Autodesk Fusion 360 part; units mm, degrees
(part 3 of 7)
  spline S687 degree 3 poles (51.2491, 62.2155) (51.339, 62.0596) (51.4081, 61.8927) (51.4547, 61.7189) knots 0 0 0 0 1 1 1 1
  spline S688 degree 3 poles (83.1324, 72.6381) (82.8108, 72.6437) (82.5167, 72.8204) (82.3608, 73.1016) knots 0 0 0 0 1 1 1 1
  spline S689 degree 3 poles (42.3721, 73.5812) (42.197, 73.8508) (42.1791, 74.1934) (42.3251, 74.4798) knots 0 0 0 0 1 1 1 1
  spline S690 degree 3 poles (108.782, 65.514) (108.9517, 65.7864) (108.9635, 66.1286) (108.813, 66.4121) knots 0 0 0 0 1 1 1 1
  spline S691 degree 3 poles (111.5839, 53.8372) (111.8201, 53.6007) (112.1405, 53.4678) (112.4748, 53.4677) knots 0 0 0 0 1 1 1 1
  spline S692 degree 3 poles (111.5839, 55.619) (111.3476, 55.3827) (111.2149, 55.0622) (111.2149, 54.7281) knots 0 0 0 0 1 1 1 1
  line L235 (43.0795, 74.9702) -> (44.388, 75.0385)
  spline S693 degree 3 poles (51.525, 61.1856) (51.525, 61.0055) (51.5014, 60.8262) (51.4547, 60.6523) knots 0 0 0 0 1 1 1 1
  line L236 (44.4665, 75.039) -> (44.4665, 75.039)
  spline S694 degree 3 poles (113.4943, 55.4686) (113.4167, 55.5755) (113.3227, 55.6695) (113.2158, 55.7471) knots 0 0 0 0 1 1 1 1
  spline S695 degree 3 poles (49.998, 63.1751) (50.172, 63.1286) (50.3391, 63.0594) (50.4951, 62.9694) knots 0 0 0 0 1 1 1 1
  spline S696 degree 3 poles (51.4547, 60.6523) (51.4081, 60.4785) (51.339, 60.3115) (51.2491, 60.1557) knots 0 0 0 0 1 1 1 1
  spline S697 degree 3 poles (51.4547, 61.7189) (51.5014, 61.5449) (51.525, 61.3656) (51.525, 61.1856) knots 0 0 0 0 1 1 1 1
  spline S698 degree 3 poles (113.6731, 55.1172) (113.6323, 55.243) (113.572, 55.3616) (113.4943, 55.4686) knots 0 0 0 0 1 1 1 1
  line L237 (112.4748, 55.9879) -> (112.4748, 55.9879)
  spline S699 degree 3 poles (45.237, 73.7316) (45.0911, 73.4449) (44.8032, 73.258) (44.482, 73.2412) knots 0 0 0 0 1 1 1 1
  line L238 (43.0826, 79.1343) -> (43.0826, 79.1343)
  spline S700 degree 3 poles (70.73, 75.2436) (71.0515, 75.2435) (71.3486, 75.072) (71.5093, 74.7935) knots 0 0 0 0 1 1 1 1
  spline S701 degree 3 poles (82.3769, 74.0013) (82.5425, 74.2768) (82.8425, 74.4431) (83.1639, 74.4375) knots 0 0 0 0 1 1 1 1
  line L239 (69.42, 75.2436) -> (69.42, 75.2436)
  spline S702 degree 3 poles (43.1741, 73.1724) (42.8529, 73.1556) (42.5472, 73.3114) (42.3721, 73.5812) knots 0 0 0 0 1 1 1 1
  line L240 (108.0518, 66.8896) -> (106.7428, 66.9356)
  spline S703 degree 3 poles (68.6407, 73.8938) (68.4801, 74.1722) (68.4801, 74.5151) (68.6407, 74.7935) knots 0 0 0 0 1 1 1 1
  spline S704 degree 3 poles (42.3251, 74.4798) (42.4709, 74.7663) (42.7585, 74.9533) (43.0795, 74.9702) knots 0 0 0 0 1 1 1 1
  spline S705 degree 3 poles (113.0685, 70.4573) (113.4027, 70.4575) (113.7232, 70.5904) (113.9594, 70.8268) knots 0 0 0 0 1 1 1 1
  spline S706 degree 3 poles (114.3284, 71.7177) (114.3283, 71.8499) (114.3073, 71.9812) (114.2664, 72.1069) knots 0 0 0 0 1 1 1 1
  spline S707 degree 3 poles (125.4285, 67.8353) (125.1002, 68.1635) (124.9158, 68.6087) (124.9159, 69.0729) knots 0 0 0 0 1 1 1 1
  spline S708 degree 3 poles (108.6016, 70.1256) (108.7576, 70.2155) (108.9011, 70.3255) (109.0285, 70.4527) knots 0 0 0 0 1 1 1 1
  line L241 (114.2307, 72.1771) -> (112.0303, 72.2541)
  spline S709 degree 3 poles (108.105, 69.9199) (108.2788, 69.9665) (108.4458, 70.0356) (108.6016, 70.1256) knots 0 0 0 0 1 1 1 1
  spline S710 degree 3 poles (109.5612, 71.3761) (109.6079, 71.5501) (109.6315, 71.7294) (109.6315, 71.9095) knots 0 0 0 0 1 1 1 1
  spline S711 degree 3 poles (109.6315, 71.9095) (109.6278, 72.0545) (109.6087, 72.1988) (109.5747, 72.3399) knots 0 0 0 0 1 1 1 1
  spline S712 degree 3 poles (112.1771, 70.8268) (112.4134, 70.5903) (112.7341, 70.4573) (113.0685, 70.4573) knots 0 0 0 0 1 1 1 1
  line L242 (109.0982, 72.3565) -> (109.1287, 73.2355)
  spline S713 degree 3 poles (102.0749, 73.3616) (101.7407, 73.3616) (101.4203, 73.2288) (101.184, 72.9926) knots 0 0 0 0 1 1 1 1
  spline S714 degree 3 poles (109.0383, 54.9198) (109.0383, 55.0999) (109.0146, 55.2792) (108.968, 55.4531) knots 0 0 0 0 1 1 1 1
  spline S715 degree 3 poles (103.3347, 72.1017) (103.3348, 72.2338) (103.314, 72.3651) (103.2733, 72.4908) knots 0 0 0 0 1 1 1 1
  line L243 (102.0749, 73.3616) -> (102.0749, 73.3616)
  spline S716 degree 3 poles (103.0944, 72.8422) (103.0166, 72.9491) (102.9225, 73.0431) (102.8154, 73.1207) knots 0 0 0 0 1 1 1 1
  spline S717 degree 3 poles (88.1264, 72.2505) (87.8053, 72.2553) (87.506, 72.0887) (87.3409, 71.8133) knots 0 0 0 0 1 1 1 1
  spline S718 degree 3 poles (108.968, 55.4531) (108.9214, 55.6269) (108.8523, 55.7939) (108.7623, 55.9497) knots 0 0 0 0 1 1 1 1
  spline S719 degree 3 poles (101.4816, 56.3719) (101.1475, 56.3719) (100.827, 56.2392) (100.5907, 56.0029) knots 0 0 0 0 1 1 1 1
  line L244 (106.9784, 56.9801) -> (106.9784, 56.9801)
  spline S720 degree 3 poles (126.6656, 67.3227) (126.2016, 67.3227) (125.7566, 67.5071) (125.4285, 67.8353) knots 0 0 0 0 1 1 1 1
  spline S721 degree 3 poles (124.9159, 69.0729) (124.9159, 69.537) (125.1003, 69.982) (125.4285, 70.3101) knots 0 0 0 0 1 1 1 1
  spline S722 degree 3 poles (101.184, 71.2103) (101.4203, 70.974) (101.7407, 70.8413) (102.0749, 70.8413) knots 0 0 0 0 1 1 1 1
  spline S723 degree 3 poles (102.4645, 73.2995) (102.3387, 73.3405) (102.2072, 73.3615) (102.0749, 73.3616) knots 0 0 0 0 1 1 1 1
  spline S724 degree 3 poles (127.9033, 67.8353) (127.575, 67.507) (127.1298, 67.3226) (126.6656, 67.3227) knots 0 0 0 0 1 1 1 1
  spline S725 degree 3 poles (100.815, 72.1017) (100.8149, 71.7674) (100.9476, 71.4467) (101.184, 71.2103) knots 0 0 0 0 1 1 1 1
  line L245 (88.0949, 70.4511) -> (89.4048, 70.4279)
  spline S726 degree 3 poles (107.5717, 73.9693) (107.0253, 73.9694) (106.5013, 73.7525) (106.1149, 73.3662) knots 0 0 0 0 1 1 1 1
  spline S727 degree 3 poles (102.9658, 71.2103) (103.2022, 71.4467) (103.3349, 71.7674) (103.3347, 72.1017) knots 0 0 0 0 1 1 1 1
  spline S728 degree 3 poles (106.1149, 73.3662) (105.7287, 72.9798) (105.5118, 72.4558) (105.5119, 71.9095) knots 0 0 0 0 1 1 1 1
  spline S729 degree 3 poles (87.3409, 71.8133) (87.176, 71.5381) (87.1701, 71.1959) (87.3254, 70.9152) knots 0 0 0 0 1 1 1 1
  spline S730 degree 3 poles (102.8154, 73.1207) (102.7085, 73.1984) (102.5901, 73.2587) (102.4645, 73.2995) knots 0 0 0 0 1 1 1 1
  spline S731 degree 3 poles (87.3254, 70.9152) (87.4808, 70.6344) (87.774, 70.4576) (88.0949, 70.4511) knots 0 0 0 0 1 1 1 1
  spline S732 degree 3 poles (108.968, 54.3865) (109.0146, 54.5604) (109.0383, 54.7397) (109.0383, 54.9198) knots 0 0 0 0 1 1 1 1
  line L246 (126.6656, 70.8227) -> (126.6656, 70.8227)
  spline S733 degree 3 poles (114.2664, 72.1069) (114.2552, 72.1306) (114.2433, 72.1541) (114.2307, 72.1771) knots 0 0 0 0 1 1 1 1
  spline S734 degree 3 poles (102.0749, 70.8413) (102.409, 70.8413) (102.7295, 70.974) (102.9658, 71.2103) knots 0 0 0 0 1 1 1 1
  spline S735 degree 3 poles (109.3556, 70.8795) (109.4455, 71.0354) (109.5147, 71.2023) (109.5612, 71.3761) knots 0 0 0 0 1 1 1 1
  line L247 (89.4359, 72.2278) -> (88.1264, 72.2505)
  spline S736 degree 3 poles (90.2058, 71.7637) (90.0503, 72.0447) (89.7569, 72.2215) (89.4359, 72.2278) knots 0 0 0 0 1 1 1 1
  spline S737 degree 3 poles (89.4048, 70.4279) (89.7257, 70.4232) (90.0248, 70.5898) (90.1898, 70.8651) knots 0 0 0 0 1 1 1 1
  spline S738 degree 3 poles (108.105, 73.8995) (107.931, 73.946) (107.7517, 73.9694) (107.5717, 73.9693) knots 0 0 0 0 1 1 1 1
  spline S739 degree 3 poles (101.184, 72.9926) (100.9477, 72.7563) (100.815, 72.4358) (100.815, 72.1017) knots 0 0 0 0 1 1 1 1
  spline S740 degree 3 poles (113.9594, 70.8268) (114.1957, 71.0631) (114.3284, 71.3836) (114.3284, 71.7177) knots 0 0 0 0 1 1 1 1
  line L248 (109.5747, 72.3399) -> (109.0982, 72.3565)
  spline S741 degree 3 poles (103.2733, 72.4908) (103.2325, 72.6166) (103.1721, 72.7352) (103.0944, 72.8422) knots 0 0 0 0 1 1 1 1
  spline S742 degree 3 poles (108.0084, 56.7037) (107.8525, 56.7938) (107.6856, 56.8631) (107.5118, 56.9099) knots 0 0 0 0 1 1 1 1
  spline S743 degree 3 poles (128.4159, 69.0729) (128.4159, 68.6087) (128.2315, 68.1635) (127.9033, 67.8353) knots 0 0 0 0 1 1 1 1
  spline S744 degree 3 poles (125.4285, 70.3101) (125.7566, 70.6382) (126.2016, 70.8226) (126.6656, 70.8227) knots 0 0 0 0 1 1 1 1
  spline S745 degree 3 poles (90.1898, 70.8651) (90.3551, 71.1403) (90.3612, 71.4828) (90.2058, 71.7637) knots 0 0 0 0 1 1 1 1
  spline S746 degree 3 poles (101.0258, 68.7856) (100.8557, 68.5131) (100.8437, 68.1707) (100.9943, 67.887) knots 0 0 0 0 1 1 1 1
  spline S747 degree 3 poles (101.8191, 69.2088) (101.4981, 69.2194) (101.1958, 69.0581) (101.0258, 68.7856) knots 0 0 0 0 1 1 1 1
  spline S748 degree 3 poles (108.4352, 56.3766) (108.3078, 56.5038) (108.1643, 56.6137) (108.0084, 56.7037) knots 0 0 0 0 1 1 1 1
  spline S749 degree 3 poles (109.0285, 70.4527) (109.1557, 70.5801) (109.2656, 70.7236) (109.3556, 70.8795) knots 0 0 0 0 1 1 1 1
  spline S750 degree 3 poles (100.9943, 67.887) (101.145, 67.6035) (101.4352, 67.4218) (101.756, 67.41) knots 0 0 0 0 1 1 1 1
  spline S751 degree 3 poles (109.0285, 73.3662) (108.9011, 73.4934) (108.7576, 73.6034) (108.6016, 73.6933) knots 0 0 0 0 1 1 1 1
  spline S752 degree 3 poles (106.1149, 70.4527) (106.5013, 70.0664) (107.0253, 69.8495) (107.5717, 69.8496) knots 0 0 0 0 1 1 1 1
  spline S753 degree 3 poles (107.5118, 56.9099) (107.3378, 56.9565) (107.1585, 56.9801) (106.9784, 56.9801) knots 0 0 0 0 1 1 1 1
  spline S754 degree 3 poles (111.8081, 71.7177) (111.8081, 71.3836) (111.9408, 71.0631) (112.1771, 70.8268) knots 0 0 0 0 1 1 1 1
  spline S755 degree 3 poles (108.7623, 55.9497) (108.6724, 56.1057) (108.5624, 56.2492) (108.4352, 56.3766) knots 0 0 0 0 1 1 1 1
  spline S756 degree 3 poles (108.6016, 73.6933) (108.4458, 73.7835) (108.2788, 73.8528) (108.105, 73.8995) knots 0 0 0 0 1 1 1 1
  spline S757 degree 3 poles (112.0303, 72.2541) (111.9155, 72.0951) (111.8394, 71.9114) (111.8081, 71.7177) knots 0 0 0 0 1 1 1 1
  spline S758 degree 3 poles (105.5119, 71.9095) (105.5118, 71.3631) (105.7287, 70.8391) (106.1149, 70.4527) knots 0 0 0 0 1 1 1 1
  spline S759 degree 3 poles (109.1287, 73.2355) (109.097, 73.2804) (109.0636, 73.324) (109.0285, 73.3662) knots 0 0 0 0 1 1 1 1
  spline S760 degree 3 poles (107.5717, 69.8496) (107.7518, 69.8496) (107.9311, 69.8733) (108.105, 69.9199) knots 0 0 0 0 1 1 1 1
  spline S761 degree 3 poles (99.6285, 38.1224) (99.6285, 38.4565) (99.7612, 38.777) (99.9975, 39.0133) knots 0 0 0 0 1 1 1 1
  spline S762 degree 3 poles (52.0955, 38.372) (52.1288, 38.5277) (52.1203, 38.6894) (52.0707, 38.8407) knots 0 0 0 0 1 1 1 1
  spline S763 degree 3 poles (105.918, 65.6137) (106.0687, 65.3303) (106.359, 65.1485) (106.6798, 65.1367) knots 0 0 0 0 1 1 1 1
  spline S764 degree 3 poles (34.5209, 42.8735) (34.5311, 42.7409) (34.5942, 42.618) (34.6961, 42.5324) knots 0 0 0 0 1 1 1 1
  line L249 (39.5454, 42.8115) -> (39.6456, 41.6658)
  line L250 (13.8684, 45.3834) -> (13.8684, 45.3834)
  spline S765 degree 3 poles (101.7793, 37.2315) (101.5431, 36.995) (101.2226, 36.8621) (100.8884, 36.862) knots 0 0 0 0 1 1 1 1
  spline S766 degree 3 poles (9.1416, 27.9669) (9.2946, 27.9668) (9.447, 27.9467) (9.5948, 27.907) knots 0 0 0 0 1 1 1 1
  spline S767 degree 3 poles (10.6572, 27.092) (10.7336, 26.9596) (10.7924, 26.8176) (10.8319, 26.6698) knots 0 0 0 0 1 1 1 1
  line L251 (51.2702, 39.25) -> (49.9623, 39.1812)
  spline S768 degree 3 poles (10.017, 27.7323) (10.1493, 27.6559) (10.2711, 27.5624) (10.3792, 27.4543) knots 0 0 0 0 1 1 1 1
  spline S769 degree 3 poles (10.8319, 26.6698) (10.8716, 26.5221) (10.8918, 26.3697) (10.8918, 26.2166) knots 0 0 0 0 1 1 1 1
  spline S770 degree 3 poles (99.9975, 39.0133) (100.2338, 39.2495) (100.5542, 39.3823) (100.8884, 39.3822) knots 0 0 0 0 1 1 1 1
  spline S771 degree 3 poles (49.2094, 38.6908) (49.1958, 38.5844) (49.2014, 38.4764) (49.2259, 38.372) knots 0 0 0 0 1 1 1 1
  spline S772 degree 3 poles (9.1416, 24.4669) (8.6775, 24.467) (8.2325, 24.6514) (7.9044, 24.9795) knots 0 0 0 0 1 1 1 1
  spline S773 degree 3 poles (7.9044, 24.9795) (7.5763, 25.3076) (7.3919, 25.7526) (7.3918, 26.2166) knots 0 0 0 0 1 1 1 1
  spline S774 degree 3 poles (7.3918, 26.2166) (7.3918, 26.6809) (7.5762, 27.1261) (7.9044, 27.4543) knots 0 0 0 0 1 1 1 1
  spline S775 degree 3 poles (29.0101, 30.3962) (28.8745, 30.1052) (28.5941, 29.9085) (28.2742, 29.88) knots 0 0 0 0 1 1 1 1
  line L252 (33.892, 44.3246) -> (34.4335, 43.8698)
  spline S776 degree 3 poles (100.8884, 39.3822) (101.0207, 39.3823) (101.1522, 39.3616) (101.278, 39.3208) knots 0 0 0 0 1 1 1 1
  line L253 (34.4335, 43.8698) -> (34.5209, 42.8735)
  spline S777 degree 3 poles (49.2259, 38.372) (49.2014, 38.4764) (49.1958, 38.5844) (49.2094, 38.6908) knots 0 0 0 0 1 1 1 1
  spline S778 degree 3 poles (103.0655, 67.364) (103.3863, 67.3536) (103.6884, 67.5149) (103.8582, 67.7872) knots 0 0 0 0 1 1 1 1
  spline S779 degree 3 poles (34.6961, 42.5324) (34.798, 42.447) (34.9301, 42.4062) (35.0624, 42.4193) knots 0 0 0 0 1 1 1 1
  spline S780 degree 3 poles (51.2702, 39.25) (51.591, 39.2661) (51.896, 39.1101) (52.0707, 38.8407) knots 0 0 0 0 1 1 1 1
  spline S781 degree 3 poles (49.2094, 38.6908) (49.355, 38.9768) (49.6418, 39.1637) (49.9623, 39.1812) knots 0 0 0 0 1 1 1 1
  spline S782 degree 3 poles (10.8918, 26.2166) (10.8917, 25.7526) (10.7073, 25.3076) (10.3792, 24.9795) knots 0 0 0 0 1 1 1 1
  spline S783 degree 3 poles (102.1483, 38.1224) (102.1483, 37.7882) (102.0155, 37.4678) (101.7793, 37.2315) knots 0 0 0 0 1 1 1 1
  spline S784 degree 3 poles (10.3792, 24.9795) (10.051, 24.6512) (9.6058, 24.4668) (9.1416, 24.4669) knots 0 0 0 0 1 1 1 1
  spline S785 degree 3 poles (101.6289, 39.1414) (101.736, 39.0638) (101.8301, 38.9698) (101.908, 38.8629) knots 0 0 0 0 1 1 1 1
  line L254 (42.2108, 41.8901) -> (42.5183, 38.372)
  spline S786 degree 3 poles (101.278, 39.3208) (101.4037, 39.2798) (101.5221, 39.2192) (101.6289, 39.1414) knots 0 0 0 0 1 1 1 1
  spline S787 degree 3 poles (7.9044, 27.4543) (8.2325, 27.7824) (8.6775, 27.9668) (9.1416, 27.9669) knots 0 0 0 0 1 1 1 1
  line L255 (28.2742, 29.88) -> (26.9694, 29.7658)
  line L256 (49.2259, 38.372) -> (52.0955, 38.372)
  spline S788 degree 3 poles (52.0707, 38.8407) (51.896, 39.1101) (51.591, 39.2661) (51.2702, 39.25) knots 0 0 0 0 1 1 1 1
  spline S789 degree 3 poles (28.1962, 31.6763) (28.4894, 31.6758) (28.764, 31.5325) (28.9321, 31.2923) knots 0 0 0 0 1 1 1 1
  spline S790 degree 3 poles (99.9975, 37.2315) (99.7612, 37.4678) (99.6285, 37.7882) (99.6285, 38.1224) knots 0 0 0 0 1 1 1 1
  spline S791 degree 3 poles (28.9321, 31.2923) (29.1162, 31.029) (29.1459, 30.6874) (29.0101, 30.3962) knots 0 0 0 0 1 1 1 1
  spline S792 degree 3 poles (26.1545, 30.1461) (25.9702, 30.4094) (25.9403, 30.7509) (26.0759, 31.0422) knots 0 0 0 0 1 1 1 1
  spline S793 degree 3 poles (28.1177, 31.6732) (28.1438, 31.6753) (28.17, 31.6764) (28.1962, 31.6763) knots 0 0 0 0 1 1 1 1
  spline S794 degree 3 poles (106.7428, 66.9356) (106.4218, 66.9462) (106.1195, 66.7849) (105.9496, 66.5124) knots 0 0 0 0 1 1 1 1
  line L257 (103.128, 69.1628) -> (101.8191, 69.2088)
  spline S795 degree 3 poles (14.7614, 44.1065) (14.897, 44.3978) (14.8671, 44.7393) (14.6828, 45.0026) knots 0 0 0 0 1 1 1 1
  spline S796 degree 3 poles (14.6828, 45.0026) (14.4987, 45.2657) (14.1884, 45.4109) (13.8684, 45.3834) knots 0 0 0 0 1 1 1 1
  spline S797 degree 3 poles (26.9694, 29.7658) (26.6493, 29.738) (26.3388, 29.883) (26.1545, 30.1461) knots 0 0 0 0 1 1 1 1
  line L258 (35.0624, 42.4193) -> (39.5454, 42.8115)
  line L259 (100.8884, 39.3822) -> (100.8884, 39.3822)
  line L260 (106.6798, 65.1367) -> (107.9887, 65.0907)
  spline S798 degree 3 poles (10.3792, 27.4543) (10.4873, 27.3462) (10.5808, 27.2244) (10.6572, 27.092) knots 0 0 0 0 1 1 1 1
  line L261 (9.1416, 27.9669) -> (9.1416, 27.9669)
  spline S799 degree 3 poles (105.9496, 66.5124) (105.7795, 66.2399) (105.7674, 65.8974) (105.918, 65.6137) knots 0 0 0 0 1 1 1 1
  spline S800 degree 3 poles (9.5948, 27.907) (9.7425, 27.8675) (9.8845, 27.8087) (10.017, 27.7323) knots 0 0 0 0 1 1 1 1
  spline S801 degree 3 poles (103.8898, 68.6854) (103.7392, 68.969) (103.4489, 69.151) (103.128, 69.1628) knots 0 0 0 0 1 1 1 1
  line L262 (5.5077, 35.7706) -> (5.5077, 35.7706)
  spline S802 degree 3 poles (101.908, 38.8629) (101.9856, 38.7559) (102.046, 38.6373) (102.0868, 38.5115) knots 0 0 0 0 1 1 1 1
  spline S803 degree 3 poles (103.8582, 67.7872) (104.0282, 68.0596) (104.0402, 68.4018) (103.8898, 68.6854) knots 0 0 0 0 1 1 1 1
  line L263 (101.756, 67.41) -> (103.0655, 67.364)
  spline S804 degree 3 poles (49.9623, 39.1812) (49.6418, 39.1637) (49.355, 38.9768) (49.2094, 38.6908) knots 0 0 0 0 1 1 1 1
  line L264 (39.6456, 41.6658) -> (42.2108, 41.8901)
  line L265 (49.9623, 39.1812) -> (51.2702, 39.25)
  spline S805 degree 3 poles (100.8884, 36.862) (100.5542, 36.8621) (100.2337, 36.995) (99.9975, 37.2315) knots 0 0 0 0 1 1 1 1
  line L266 (42.5183, 38.372) -> (49.2259, 38.372)
  spline S806 degree 3 poles (102.0868, 38.5115) (102.1275, 38.3858) (102.1483, 38.2545) (102.1483, 38.1224) knots 0 0 0 0 1 1 1 1
  spline S807 degree 3 poles (26.7141, 33.2012) (26.38, 33.2012) (26.0595, 33.3339) (25.8232, 33.5702) knots 0 0 0 0 1 1 1 1
  line L267 (106.8022, 31.1114) -> (105.4933, 31.1574)
  spline S808 degree 3 poles (25.8232, 35.352) (26.0594, 35.5884) (26.3799, 35.7214) (26.7141, 35.7215) knots 0 0 0 0 1 1 1 1
  spline S809 degree 3 poles (7.0233, 34.8957) (7.0998, 34.7632) (7.1585, 34.6213) (7.198, 34.4735) knots 0 0 0 0 1 1 1 1
  spline S810 degree 3 poles (7.198, 34.4735) (7.2377, 34.3259) (7.2578, 34.1737) (7.258, 34.0208) knots 0 0 0 0 1 1 1 1
  spline S811 degree 3 poles (6.7453, 32.7832) (6.417, 32.4551) (5.9718, 32.2709) (5.5077, 32.2711) knots 0 0 0 0 1 1 1 1
  spline S812 degree 3 poles (100.5695, 33.4307) (100.2487, 33.4424) (99.9585, 33.6242) (99.8078, 33.9076) knots 0 0 0 0 1 1 1 1
  line L268 (100.6321, 35.2295) -> (100.6321, 35.2295)
  spline S813 degree 3 poles (3.7579, 34.0208) (3.7579, 34.485) (3.9423, 34.9302) (4.2705, 35.2585) knots 0 0 0 0 1 1 1 1
  spline S814 degree 3 poles (98.6616, 20.925) (98.8355, 20.8784) (99.0024, 20.8093) (99.1583, 20.7193) knots 0 0 0 0 1 1 1 1
  spline S815 degree 3 poles (68.7818, 18.5267) (68.7818, 18.9909) (68.9662, 19.4361) (69.2945, 19.7643) knots 0 0 0 0 1 1 1 1
  spline S816 degree 3 poles (99.1583, 20.7193) (99.3142, 20.6294) (99.4577, 20.5194) (99.5851, 20.3922) knots 0 0 0 0 1 1 1 1
  spline S817 degree 3 poles (102.6717, 33.8079) (102.5018, 33.5354) (102.1995, 33.3741) (101.8785, 33.3847) knots 0 0 0 0 1 1 1 1
  line L269 (26.8123, 31.559) -> (28.1177, 31.6732)
  spline S818 degree 3 poles (26.7141, 35.7215) (26.8465, 35.7214) (26.9779, 35.7005) (27.1038, 35.6595) knots 0 0 0 0 1 1 1 1
  line L270 (26.7141, 35.7215) -> (26.7141, 35.7215)
  spline S819 degree 3 poles (25.4543, 34.4611) (25.4542, 34.7952) (25.587, 35.1157) (25.8232, 35.352) knots 0 0 0 0 1 1 1 1
  line L271 (105.5558, 32.9563) -> (106.8653, 32.9103)
  spline S820 degree 3 poles (104.7626, 32.5331) (104.9325, 32.8056) (105.2348, 32.9668) (105.5558, 32.9563) knots 0 0 0 0 1 1 1 1
  spline S821 degree 3 poles (7.258, 34.0208) (7.258, 33.5566) (7.0736, 33.1114) (6.7453, 32.7832) knots 0 0 0 0 1 1 1 1
  spline S822 degree 3 poles (99.8394, 34.8063) (100.0092, 35.0786) (100.3113, 35.2399) (100.6321, 35.2295) knots 0 0 0 0 1 1 1 1
  spline S823 degree 3 poles (5.5077, 32.2711) (5.0437, 32.271) (4.5987, 32.4552) (4.2705, 32.7832) knots 0 0 0 0 1 1 1 1
  spline S824 degree 3 poles (27.1038, 35.6595) (27.2294, 35.6186) (27.3478, 35.5583) (27.4546, 35.4807) knots 0 0 0 0 1 1 1 1
  spline S825 degree 3 poles (27.974, 34.4611) (27.974, 34.329) (27.9533, 34.1977) (27.9125, 34.072) knots 0 0 0 0 1 1 1 1
  spline S826 degree 3 poles (5.9609, 35.7112) (6.1085, 35.6716) (6.2502, 35.6129) (6.3826, 35.5365) knots 0 0 0 0 1 1 1 1
  spline S827 degree 3 poles (4.2705, 32.7832) (3.9423, 33.1114) (3.7579, 33.5566) (3.7579, 34.0208) knots 0 0 0 0 1 1 1 1
  spline S828 degree 3 poles (102.7033, 34.706) (102.8537, 34.4225) (102.8417, 34.0802) (102.6717, 33.8079) knots 0 0 0 0 1 1 1 1
  line L272 (105.5558, 32.9563) -> (105.5558, 32.9563)
  spline S829 degree 3 poles (69.2945, 19.7643) (69.6226, 20.0925) (70.0676, 20.2769) (70.5316, 20.277) knots 0 0 0 0 1 1 1 1
  spline S830 degree 3 poles (25.8232, 33.5702) (25.587, 33.8065) (25.4542, 34.127) (25.4543, 34.4611) knots 0 0 0 0 1 1 1 1
  spline S831 degree 3 poles (27.4546, 35.4807) (27.5617, 35.4029) (27.6559, 35.3087) (27.7337, 35.2016) knots 0 0 0 0 1 1 1 1
  spline S832 degree 3 poles (101.9416, 35.1835) (102.2625, 35.1717) (102.5527, 34.9897) (102.7033, 34.706) knots 0 0 0 0 1 1 1 1
  spline S833 degree 3 poles (5.5077, 35.7706) (5.6607, 35.7707) (5.8131, 35.7507) (5.9609, 35.7112) knots 0 0 0 0 1 1 1 1
  spline S834 degree 3 poles (4.2705, 35.2585) (4.5987, 35.5864) (5.0437, 35.7706) (5.5077, 35.7706) knots 0 0 0 0 1 1 1 1
  line L273 (70.5316, 20.277) -> (70.5316, 20.277)
  spline S835 degree 3 poles (27.7337, 35.2016) (27.8113, 35.0948) (27.8717, 34.9764) (27.9125, 34.8507) knots 0 0 0 0 1 1 1 1
  spline S836 degree 3 poles (27.7337, 33.7206) (27.6559, 33.6137) (27.5617, 33.5197) (27.4546, 33.442) knots 0 0 0 0 1 1 1 1
  spline S837 degree 3 poles (107.6285, 32.4333) (107.7793, 32.1495) (107.7673, 31.8067) (107.597, 31.5342) knots 0 0 0 0 1 1 1 1
  spline S838 degree 3 poles (99.5851, 20.3922) (99.7123, 20.2648) (99.8223, 20.1213) (99.9122, 19.9654) knots 0 0 0 0 1 1 1 1
  spline S839 degree 3 poles (100.1184, 19.4687) (100.1649, 19.2948) (100.1883, 19.1155) (100.1882, 18.9354) knots 0 0 0 0 1 1 1 1
  spline S840 degree 3 poles (100.1184, 18.4021) (100.0717, 18.2283) (100.0023, 18.0613) (99.9122, 17.9055) knots 0 0 0 0 1 1 1 1
  spline S841 degree 3 poles (98.1283, 20.9953) (98.3084, 20.9952) (98.4877, 20.9716) (98.6616, 20.925) knots 0 0 0 0 1 1 1 1
  spline S842 degree 3 poles (99.9122, 17.9055) (99.8223, 17.7496) (99.7123, 17.6061) (99.5851, 17.4787) knots 0 0 0 0 1 1 1 1
  spline S843 degree 3 poles (99.5851, 17.4787) (99.4577, 17.3515) (99.3142, 17.2415) (99.1583, 17.1516) knots 0 0 0 0 1 1 1 1
  spline S844 degree 3 poles (26.0759, 31.0422) (26.2115, 31.3336) (26.4922, 31.5305) (26.8123, 31.559) knots 0 0 0 0 1 1 1 1
  spline S845 degree 3 poles (98.6616, 16.9454) (98.4877, 16.8987) (98.3084, 16.8751) (98.1283, 16.8751) knots 0 0 0 0 1 1 1 1
  spline S846 degree 3 poles (99.1583, 17.1516) (99.0024, 17.0614) (98.8355, 16.9921) (98.6616, 16.9454) knots 0 0 0 0 1 1 1 1
  line L274 (100.6321, 35.2295) -> (101.9416, 35.1835)
  spline S847 degree 3 poles (27.4546, 33.442) (27.3478, 33.3642) (27.2294, 33.3037) (27.1038, 33.2627) knots 0 0 0 0 1 1 1 1
  spline S848 degree 3 poles (99.9122, 19.9654) (100.0023, 19.8095) (100.0717, 19.6426) (100.1184, 19.4687) knots 0 0 0 0 1 1 1 1
  spline S849 degree 3 poles (100.1882, 18.9354) (100.1883, 18.7554) (100.1649, 18.5761) (100.1184, 18.4021) knots 0 0 0 0 1 1 1 1
  spline S850 degree 3 poles (27.9125, 34.072) (27.8717, 33.9462) (27.8114, 33.8276) (27.7337, 33.7206) knots 0 0 0 0 1 1 1 1
  spline S851 degree 3 poles (99.8078, 33.9076) (99.6572, 34.1914) (99.6692, 34.5338) (99.8394, 34.8063) knots 0 0 0 0 1 1 1 1
  spline S852 degree 3 poles (27.9125, 34.8507) (27.9533, 34.7249) (27.9741, 34.5934) (27.974, 34.4611) knots 0 0 0 0 1 1 1 1
  spline S853 degree 3 poles (98.1283, 16.8751) (97.5819, 16.8751) (97.0579, 17.0922) (96.6716, 17.4787) knots 0 0 0 0 1 1 1 1
  spline S854 degree 3 poles (107.597, 31.5342) (107.4267, 31.2614) (107.1237, 31.1002) (106.8022, 31.1114) knots 0 0 0 0 1 1 1 1
  spline S855 degree 3 poles (105.4933, 31.1574) (105.1725, 31.1692) (104.8822, 31.3509) (104.7316, 31.6344) knots 0 0 0 0 1 1 1 1
  spline S856 degree 3 poles (6.3826, 35.5365) (6.5151, 35.4601) (6.6371, 35.3666) (6.7453, 35.2585) knots 0 0 0 0 1 1 1 1
  spline S857 degree 3 poles (6.7453, 35.2585) (6.8535, 35.1502) (6.9469, 35.0283) (7.0233, 34.8957) knots 0 0 0 0 1 1 1 1
  line L275 (101.8785, 33.3847) -> (100.5695, 33.4307)
  line L276 (28.1962, 31.6763) -> (28.1962, 31.6763)
  spline S858 degree 3 poles (104.7316, 31.6344) (104.5808, 31.918) (104.5926, 32.2605) (104.7626, 32.5331) knots 0 0 0 0 1 1 1 1
  spline S859 degree 3 poles (27.1038, 33.2627) (26.9779, 33.2219) (26.8464, 33.2011) (26.7141, 33.2012) knots 0 0 0 0 1 1 1 1
  spline S860 degree 3 poles (106.8653, 32.9103) (107.1866, 32.8991) (107.4776, 32.7172) (107.6285, 32.4333) knots 0 0 0 0 1 1 1 1
  spline S861 degree 3 poles (110.1416, 22.527) (110.2946, 22.5269) (110.447, 22.5067) (110.5948, 22.467) knots 0 0 0 0 1 1 1 1
  spline S862 degree 3 poles (111.8319, 21.2299) (111.8716, 21.0821) (111.8918, 20.9297) (111.8918, 20.7767) knots 0 0 0 0 1 1 1 1
  spline S863 degree 3 poles (93.9276, 19.5953) (93.8868, 19.4696) (93.8264, 19.351) (93.7488, 19.2439) knots 0 0 0 0 1 1 1 1
  line L277 (92.7292, 21.2449) -> (92.7292, 21.2449)
  spline S864 degree 3 poles (34.0961, 29.6361) (34.2802, 29.3727) (34.3099, 29.0312) (34.1741, 28.74) knots 0 0 0 0 1 1 1 1
  spline S865 degree 3 poles (32.1334, 28.1096) (31.813, 28.0814) (31.5019, 28.2264) (31.3175, 28.4899) knots 0 0 0 0 1 1 1 1
  line L278 (33.3602, 30.02) -> (33.3602, 30.02)
  spline S866 degree 3 poles (36.7812, 34.5288) (37.0175, 34.2925) (37.338, 34.1598) (37.6721, 34.1598) knots 0 0 0 0 1 1 1 1
  spline S867 degree 3 poles (36.5807, 35.8264) (36.5012, 35.7019) (36.4441, 35.5644) (36.4122, 35.4202) knots 0 0 0 0 1 1 1 1
  spline S868 degree 3 poles (38.9325, 35.4202) (38.9324, 35.5524) (38.9114, 35.6837) (38.8705, 35.8093) knots 0 0 0 0 1 1 1 1
  spline S869 degree 3 poles (38.8705, 35.8093) (38.8417, 35.8819) (38.8062, 35.9516) (38.7645, 36.0176) knots 0 0 0 0 1 1 1 1
  spline S870 degree 3 poles (32.7262, 36.9302) (32.5524, 36.9768) (32.3733, 37.0004) (32.1934, 37.0005) knots 0 0 0 0 1 1 1 1
  spline S871 degree 3 poles (33.2233, 36.7245) (33.0673, 36.8145) (32.9001, 36.8837) (32.7262, 36.9302) knots 0 0 0 0 1 1 1 1
  spline S872 degree 3 poles (33.5768, 36.4532) (33.4691, 36.5562) (33.3506, 36.6471) (33.2233, 36.7245) knots 0 0 0 0 1 1 1 1
  spline S873 degree 3 poles (30.133, 34.9407) (30.1331, 34.3942) (30.3502, 33.8702) (30.7366, 33.4839) knots 0 0 0 0 1 1 1 1
  line L279 (103.5275, 19.1458) -> (103.5275, 19.1458)
  spline S874 degree 3 poles (37.6721, 34.1598) (38.0063, 34.1598) (38.3267, 34.2925) (38.563, 34.5288) knots 0 0 0 0 1 1 1 1
  spline S875 degree 3 poles (93.7488, 20.7255) (93.8264, 20.6185) (93.8868, 20.4999) (93.9276, 20.3741) knots 0 0 0 0 1 1 1 1
  line L280 (98.1283, 20.9953) -> (98.1283, 20.9953)
  spline S876 degree 3 poles (93.9896, 19.985) (93.9895, 19.8527) (93.9686, 19.7212) (93.9276, 19.5953) knots 0 0 0 0 1 1 1 1
  spline S877 degree 3 poles (93.9276, 20.3741) (93.9685, 20.2485) (93.9894, 20.1171) (93.9896, 19.985) knots 0 0 0 0 1 1 1 1
  spline S878 degree 3 poles (93.7488, 19.2439) (93.6711, 19.1371) (93.5771, 19.0431) (93.4702, 18.9654) knots 0 0 0 0 1 1 1 1
  spline S879 degree 3 poles (92.7292, 18.7246) (92.3951, 18.7246) (92.0746, 18.8573) (91.8383, 19.0936) knots 0 0 0 0 1 1 1 1
  spline S880 degree 3 poles (93.1188, 21.1834) (93.2447, 21.1424) (93.3632, 21.0819) (93.4702, 21.004) knots 0 0 0 0 1 1 1 1
  spline S881 degree 3 poles (93.4702, 18.9654) (93.3632, 18.8877) (93.2446, 18.8274) (93.1188, 18.7866) knots 0 0 0 0 1 1 1 1
  spline S882 degree 3 poles (91.8383, 20.8759) (92.0746, 21.1121) (92.3951, 21.2449) (92.7292, 21.2449) knots 0 0 0 0 1 1 1 1
  spline S883 degree 3 poles (111.017, 22.2923) (111.1493, 22.2159) (111.2711, 22.1224) (111.3792, 22.0143) knots 0 0 0 0 1 1 1 1
  spline S884 degree 3 poles (111.3792, 22.0143) (111.4873, 21.9061) (111.5808, 21.7841) (111.6572, 21.6516) knots 0 0 0 0 1 1 1 1
  spline S885 degree 3 poles (33.2817, 30.0169) (33.3078, 30.0191) (33.334, 30.0201) (33.3602, 30.02) knots 0 0 0 0 1 1 1 1
  line L281 (38.7645, 36.0176) -> (36.5807, 35.8264)
  spline S886 degree 3 poles (31.3175, 28.4899) (31.1332, 28.7534) (31.1034, 29.0951) (31.2394, 29.3865) knots 0 0 0 0 1 1 1 1
  spline S887 degree 3 poles (102.6366, 18.7768) (102.8729, 19.013) (103.1934, 19.1458) (103.5275, 19.1458) knots 0 0 0 0 1 1 1 1
  line L282 (110.1416, 22.527) -> (110.1416, 22.527)
  spline S888 degree 3 poles (70.5316, 20.277) (70.6846, 20.2769) (70.837, 20.2567) (70.9848, 20.217) knots 0 0 0 0 1 1 1 1
  spline S889 degree 3 poles (71.4065, 20.0423) (71.539, 19.9659) (71.661, 19.8725) (71.7692, 19.7643) knots 0 0 0 0 1 1 1 1
  spline S890 degree 3 poles (30.7366, 33.4839) (31.123, 33.0977) (31.647, 32.8807) (32.1934, 32.8808) knots 0 0 0 0 1 1 1 1
  spline S891 degree 3 poles (36.4122, 35.4202) (36.4121, 35.0859) (36.5448, 34.7652) (36.7812, 34.5288) knots 0 0 0 0 1 1 1 1
  spline S892 degree 3 poles (110.1416, 19.0269) (109.6775, 19.027) (109.2325, 19.2114) (108.9044, 19.5395) knots 0 0 0 0 1 1 1 1
  spline S893 degree 3 poles (108.9044, 19.5395) (108.5763, 19.8676) (108.3919, 20.3126) (108.3918, 20.7767) knots 0 0 0 0 1 1 1 1
  spline S894 degree 3 poles (38.563, 34.5288) (38.7996, 34.7651) (38.9325, 35.0858) (38.9325, 35.4202) knots 0 0 0 0 1 1 1 1
  spline S895 degree 3 poles (32.7262, 32.9506) (32.9002, 32.9973) (33.0673, 33.0666) (33.2233, 33.1568) knots 0 0 0 0 1 1 1 1
  spline S896 degree 3 poles (31.2394, 29.3865) (31.3752, 29.6778) (31.6561, 29.8746) (31.9763, 29.9027) knots 0 0 0 0 1 1 1 1
  spline S897 degree 3 poles (91.4693, 19.985) (91.4693, 20.3191) (91.602, 20.6396) (91.8383, 20.8759) knots 0 0 0 0 1 1 1 1
  spline S898 degree 3 poles (111.6572, 21.6516) (111.7336, 21.5192) (111.7923, 21.3775) (111.8319, 21.2299) knots 0 0 0 0 1 1 1 1
  spline S899 degree 3 poles (32.1934, 37.0005) (31.647, 37.0006) (31.123, 36.7837) (30.7366, 36.3974) knots 0 0 0 0 1 1 1 1
  spline S900 degree 3 poles (96.6716, 17.4787) (96.2853, 17.8651) (96.0684, 18.3891) (96.0685, 18.9354) knots 0 0 0 0 1 1 1 1
  spline S901 degree 3 poles (93.4702, 21.004) (93.5771, 20.9264) (93.6711, 20.8324) (93.7488, 20.7255) knots 0 0 0 0 1 1 1 1
  spline S902 degree 3 poles (93.1188, 18.7866) (92.993, 18.7456) (92.8615, 18.7247) (92.7292, 18.7246) knots 0 0 0 0 1 1 1 1
  spline S903 degree 3 poles (110.5948, 22.467) (110.7425, 22.4275) (110.8845, 22.3688) (111.017, 22.2923) knots 0 0 0 0 1 1 1 1
  spline S904 degree 3 poles (102.2671, 17.8859) (102.2672, 18.2201) (102.4002, 18.5406) (102.6366, 18.7768) knots 0 0 0 0 1 1 1 1
  spline S905 degree 3 poles (32.1934, 32.8808) (32.3733, 32.8807) (32.5524, 32.9042) (32.7262, 32.9506) knots 0 0 0 0 1 1 1 1
  spline S906 degree 3 poles (96.0685, 18.9354) (96.0684, 19.4818) (96.2853, 20.0058) (96.6716, 20.3922) knots 0 0 0 0 1 1 1 1
  spline S907 degree 3 poles (111.3792, 19.5395) (111.051, 19.2113) (110.6058, 19.0269) (110.1416, 19.0269) knots 0 0 0 0 1 1 1 1
  spline S908 degree 3 poles (108.3918, 20.7767) (108.3918, 21.2409) (108.5762, 21.6861) (108.9044, 22.0143) knots 0 0 0 0 1 1 1 1
  spline S909 degree 3 poles (30.7366, 36.3974) (30.3502, 36.0111) (30.1331, 35.4871) (30.133, 34.9407) knots 0 0 0 0 1 1 1 1
  spline S910 degree 3 poles (34.1741, 28.74) (34.0385, 28.449) (33.7581, 28.2523) (33.4383, 28.2238) knots 0 0 0 0 1 1 1 1
  spline S911 degree 3 poles (92.7292, 21.2449) (92.8615, 21.2449) (92.993, 21.2242) (93.1188, 21.1834) knots 0 0 0 0 1 1 1 1
  spline S912 degree 3 poles (111.8918, 20.7767) (111.8917, 20.3126) (111.7074, 19.8676) (111.3792, 19.5395) knots 0 0 0 0 1 1 1 1
  spline S913 degree 3 poles (96.6716, 20.3922) (97.058, 20.7784) (97.582, 20.9954) (98.1283, 20.9953) knots 0 0 0 0 1 1 1 1
  spline S914 degree 3 poles (108.9044, 22.0143) (109.2325, 22.3425) (109.6775, 22.5269) (110.1416, 22.527) knots 0 0 0 0 1 1 1 1
  spline S915 degree 3 poles (91.8383, 19.0936) (91.6019, 19.33) (91.4692, 19.6507) (91.4693, 19.985) knots 0 0 0 0 1 1 1 1
  line L283 (33.4383, 28.2238) -> (32.1334, 28.1096)
  spline S916 degree 3 poles (33.3602, 30.02) (33.6534, 30.0195) (33.928, 29.8763) (34.0961, 29.6361) knots 0 0 0 0 1 1 1 1
  line L284 (31.9763, 29.9027) -> (33.2817, 30.0169)
  spline S917 degree 3 poles (87.1151, 58.7842) (87.5015, 58.3979) (88.0255, 58.181) (88.5718, 58.1811) knots 0 0 0 0 1 1 1 1
  spline S918 degree 3 poles (90.6316, 60.2409) (90.6316, 60.421) (90.608, 60.6003) (90.5614, 60.7742) knots 0 0 0 0 1 1 1 1
  spline S919 degree 3 poles (84.9462, 56.9533) (85.1017, 56.6724) (85.0958, 56.33) (84.9307, 56.0546) knots 0 0 0 0 1 1 1 1
  spline S920 degree 3 poles (82.0642, 56.1042) (81.9085, 56.3855) (81.9146, 56.7284) (82.0802, 57.0039) knots 0 0 0 0 1 1 1 1
  spline S921 degree 3 poles (70.9848, 20.217) (71.1324, 20.1775) (71.2741, 20.1187) (71.4065, 20.0423) knots 0 0 0 0 1 1 1 1
  spline S922 degree 3 poles (90.0286, 61.6977) (90.1558, 61.5703) (90.2658, 61.4268) (90.3557, 61.2708) knots 0 0 0 0 1 1 1 1
  spline S923 degree 3 poles (72.0473, 19.4016) (72.1236, 19.2692) (72.1824, 19.1275) (72.2219, 18.9799) knots 0 0 0 0 1 1 1 1
  spline S924 degree 3 poles (89.6017, 62.0248) (89.4459, 62.1149) (89.279, 62.1842) (89.1051, 62.231) knots 0 0 0 0 1 1 1 1
  spline S925 degree 3 poles (89.6017, 62.0248) (89.7577, 61.9349) (89.9012, 61.8249) (90.0286, 61.6977) knots 0 0 0 0 1 1 1 1
  spline S926 degree 3 poles (90.0286, 58.7842) (90.1558, 58.9115) (90.2658, 59.055) (90.3557, 59.211) knots 0 0 0 0 1 1 1 1
  spline S927 degree 3 poles (90.5614, 60.7742) (90.5148, 60.948) (90.4456, 61.115) (90.3557, 61.2708) knots 0 0 0 0 1 1 1 1
  spline S928 degree 3 poles (90.5614, 59.7076) (90.5148, 59.5338) (90.4456, 59.3668) (90.3557, 59.211) knots 0 0 0 0 1 1 1 1
  spline S929 degree 3 poles (84.9307, 56.0546) (84.7656, 55.7792) (84.4663, 55.6126) (84.1452, 55.6174) knots 0 0 0 0 1 1 1 1
  spline S930 degree 3 poles (72.2819, 18.5267) (72.2818, 18.0626) (72.0974, 17.6176) (71.7692, 17.2895) knots 0 0 0 0 1 1 1 1
  spline S931 degree 3 poles (90.5614, 60.7742) (90.608, 60.6003) (90.6316, 60.421) (90.6316, 60.2409) knots 0 0 0 0 1 1 1 1
  spline S932 degree 3 poles (90.3557, 59.211) (90.2658, 59.055) (90.1558, 58.9115) (90.0286, 58.7842) knots 0 0 0 0 1 1 1 1
  line L285 (84.1452, 55.6174) -> (82.8357, 55.6407)
  spline S933 degree 3 poles (90.0286, 61.6977) (89.9012, 61.8249) (89.7577, 61.9349) (89.6017, 62.0248) knots 0 0 0 0 1 1 1 1
  spline S934 degree 3 poles (87.1151, 61.6977) (86.7288, 61.3113) (86.5119, 60.7873) (86.512, 60.2409) knots 0 0 0 0 1 1 1 1
  spline S935 degree 3 poles (90.3557, 59.211) (90.4456, 59.3668) (90.5148, 59.5338) (90.5614, 59.7076) knots 0 0 0 0 1 1 1 1
  spline S936 degree 3 poles (87.1151, 61.6977) (87.5014, 62.0841) (88.0254, 62.3012) (88.5718, 62.3013) knots 0 0 0 0 1 1 1 1
  spline S937 degree 3 poles (71.7692, 19.7643) (71.8774, 19.6561) (71.9708, 19.5341) (72.0473, 19.4016) knots 0 0 0 0 1 1 1 1
  spline S938 degree 3 poles (72.2219, 18.9799) (72.2616, 18.8321) (72.2818, 18.6797) (72.2819, 18.5267) knots 0 0 0 0 1 1 1 1
  line L286 (84.1767, 57.4173) -> (82.8673, 57.4401)
  spline S939 degree 3 poles (90.5614, 59.7076) (90.608, 59.8815) (90.6316, 60.0608) (90.6316, 60.2409) knots 0 0 0 0 1 1 1 1
  spline S940 degree 3 poles (88.5718, 58.1811) (88.0255, 58.181) (87.5015, 58.3979) (87.1151, 58.7842) knots 0 0 0 0 1 1 1 1
  line L287 (88.5718, 62.3013) -> (88.5718, 62.3013)
  spline S941 degree 3 poles (82.0802, 57.0039) (82.2459, 57.2794) (82.5459, 57.4457) (82.8673, 57.4401) knots 0 0 0 0 1 1 1 1
  line L288 (82.8673, 57.4401) -> (84.1767, 57.4173)
  spline S942 degree 3 poles (89.1051, 62.231) (88.9312, 62.2776) (88.7519, 62.3012) (88.5718, 62.3013) knots 0 0 0 0 1 1 1 1
  spline S943 degree 3 poles (71.7692, 17.2895) (71.441, 16.9613) (70.9958, 16.7769) (70.5316, 16.7769) knots 0 0 0 0 1 1 1 1
  line L289 (82.8673, 57.4401) -> (82.8673, 57.4401)
  spline S944 degree 3 poles (89.6017, 58.457) (89.7577, 58.547) (89.9012, 58.6569) (90.0286, 58.7842) knots 0 0 0 0 1 1 1 1
  spline S945 degree 3 poles (82.8357, 55.6407) (82.5142, 55.6463) (82.2201, 55.823) (82.0642, 56.1042) knots 0 0 0 0 1 1 1 1
  spline S946 degree 3 poles (90.3557, 61.2708) (90.2658, 61.4268) (90.1558, 61.5703) (90.0286, 61.6977) knots 0 0 0 0 1 1 1 1
  spline S947 degree 3 poles (69.2945, 17.2895) (68.9663, 17.6176) (68.7819, 18.0626) (68.7818, 18.5267) knots 0 0 0 0 1 1 1 1
  spline S948 degree 3 poles (88.5718, 62.3013) (88.7519, 62.3012) (88.9312, 62.2776) (89.1051, 62.231) knots 0 0 0 0 1 1 1 1
  spline S949 degree 3 poles (88.5718, 58.1811) (88.7519, 58.1811) (88.9312, 58.2047) (89.1051, 58.2514) knots 0 0 0 0 1 1 1 1
  spline S950 degree 3 poles (89.1051, 58.2514) (89.2789, 58.2979) (89.4459, 58.3671) (89.6017, 58.457) knots 0 0 0 0 1 1 1 1
  spline S951 degree 3 poles (90.3557, 61.2708) (90.4456, 61.115) (90.5148, 60.948) (90.5614, 60.7742) knots 0 0 0 0 1 1 1 1
  spline S952 degree 3 poles (93.1798, 59.2539) (93.4161, 59.0176) (93.7366, 58.8849) (94.0707, 58.8849) knots 0 0 0 0 1 1 1 1
  spline S953 degree 3 poles (89.1051, 58.2514) (88.9312, 58.2047) (88.7519, 58.1811) (88.5718, 58.1811) knots 0 0 0 0 1 1 1 1
  spline S954 degree 3 poles (89.6017, 58.457) (89.4459, 58.3671) (89.2789, 58.2979) (89.1051, 58.2514) knots 0 0 0 0 1 1 1 1
  spline S955 degree 3 poles (87.1151, 58.7842) (86.7288, 59.1706) (86.5119, 59.6946) (86.512, 60.2409) knots 0 0 0 0 1 1 1 1
  spline S956 degree 3 poles (84.1767, 57.4173) (84.4976, 57.4109) (84.7908, 57.2341) (84.9462, 56.9533) knots 0 0 0 0 1 1 1 1
  spline S957 degree 3 poles (93.1798, 61.0362) (92.9434, 60.7998) (92.8107, 60.4791) (92.8108, 60.1448) knots 0 0 0 0 1 1 1 1
  spline S958 degree 3 poles (95.3311, 60.1448) (95.331, 60.2771) (95.3101, 60.4086) (95.2691, 60.5344) knots 0 0 0 0 1 1 1 1
  spline S959 degree 3 poles (95.2691, 60.5344) (95.2283, 60.6602) (95.168, 60.7788) (95.0903, 60.8858) knots 0 0 0 0 1 1 1 1
  spline S960 degree 3 poles (94.0707, 61.4052) (93.7366, 61.4052) (93.4161, 61.2725) (93.1798, 61.0362) knots 0 0 0 0 1 1 1 1
  spline S961 degree 3 poles (95.0903, 60.8858) (95.0126, 60.9927) (94.9186, 61.0867) (94.8118, 61.1644) knots 0 0 0 0 1 1 1 1
  spline S962 degree 3 poles (94.4604, 61.3432) (94.3345, 61.3842) (94.203, 61.4051) (94.0707, 61.4052) knots 0 0 0 0 1 1 1 1
  spline S963 degree 3 poles (70.5316, 16.7769) (70.0676, 16.777) (69.6226, 16.9614) (69.2945, 17.2895) knots 0 0 0 0 1 1 1 1
  spline S964 degree 3 poles (88.5718, 62.3013) (88.0254, 62.3012) (87.5014, 62.0841) (87.1151, 61.6977) knots 0 0 0 0 1 1 1 1
  spline S965 degree 3 poles (84.9462, 56.9533) (84.7908, 57.2341) (84.4976, 57.4109) (84.1767, 57.4173) knots 0 0 0 0 1 1 1 1
  spline S966 degree 3 poles (89.1051, 62.231) (89.279, 62.1842) (89.4459, 62.1149) (89.6017, 62.0248) knots 0 0 0 0 1 1 1 1
  spline S967 degree 3 poles (94.9621, 59.2539) (95.1984, 59.4902) (95.3311, 59.8107) (95.3311, 60.1448) knots 0 0 0 0 1 1 1 1
  spline S968 degree 3 poles (94.0707, 58.8849) (94.405, 58.8848) (94.7257, 59.0175) (94.9621, 59.2539) knots 0 0 0 0 1 1 1 1
  spline S969 degree 3 poles (86.512, 60.2409) (86.5119, 59.6946) (86.7288, 59.1706) (87.1151, 58.7842) knots 0 0 0 0 1 1 1 1
  spline S970 degree 3 poles (86.512, 60.2409) (86.5119, 60.7873) (86.7288, 61.3113) (87.1151, 61.6977) knots 0 0 0 0 1 1 1 1
  spline S971 degree 3 poles (92.8108, 60.1448) (92.8108, 59.8107) (92.9436, 59.4902) (93.1798, 59.2539) knots 0 0 0 0 1 1 1 1
  spline S972 degree 3 poles (94.0707, 61.4052) (94.203, 61.4051) (94.3345, 61.3842) (94.4604, 61.3432) knots 0 0 0 0 1 1 1 1
  spline S973 degree 3 poles (90.6316, 60.2409) (90.6316, 60.0608) (90.608, 59.8815) (90.5614, 59.7076) knots 0 0 0 0 1 1 1 1
  spline S974 degree 3 poles (90.0286, 58.7842) (89.9012, 58.6569) (89.7577, 58.547) (89.6017, 58.457) knots 0 0 0 0 1 1 1 1
  line L290 (88.5718, 62.3013) -> (88.5718, 62.3013)
  spline S975 degree 3 poles (82.1815, 59.4461) (81.9453, 59.6824) (81.8125, 60.0029) (81.8126, 60.337) knots 0 0 0 0 1 1 1 1
  spline S976 degree 3 poles (89.9087, 54.7663) (89.7533, 55.0471) (89.4601, 55.224) (89.1392, 55.2304) knots 0 0 0 0 1 1 1 1
  spline S977 degree 3 poles (82.1815, 61.2279) (82.4178, 61.4642) (82.7383, 61.5969) (83.0724, 61.5969) knots 0 0 0 0 1 1 1 1
  spline S978 degree 3 poles (87.0288, 53.9178) (86.8733, 54.1987) (86.8792, 54.5411) (87.0443, 54.8164) knots 0 0 0 0 1 1 1 1
  spline S979 degree 3 poles (82.0802, 57.0039) (81.9146, 56.7284) (81.9085, 56.3855) (82.0642, 56.1042) knots 0 0 0 0 1 1 1 1
  spline S980 degree 3 poles (94.8118, 61.1644) (94.9186, 61.0867) (95.0126, 60.9927) (95.0903, 60.8858) knots 0 0 0 0 1 1 1 1
  spline S981 degree 3 poles (92.8108, 60.1448) (92.8107, 60.4791) (92.9434, 60.7998) (93.1798, 61.0362) knots 0 0 0 0 1 1 1 1
  spline S982 degree 3 poles (87.0288, 53.9178) (87.1842, 53.637) (87.4773, 53.4602) (87.7982, 53.4537) knots 0 0 0 0 1 1 1 1
  spline S983 degree 3 poles (82.8673, 57.4401) (82.5459, 57.4457) (82.2459, 57.2794) (82.0802, 57.0039) knots 0 0 0 0 1 1 1 1
  spline S984 degree 3 poles (77.0718, 59.2916) (76.8743, 59.6337) (76.7704, 60.0217) (76.7705, 60.4166) knots 0 0 0 0 1 1 1 1
  spline S985 degree 3 poles (83.0724, 61.5969) (82.7383, 61.5969) (82.4178, 61.4642) (82.1815, 61.2279) knots 0 0 0 0 1 1 1 1
  spline S986 degree 3 poles (82.1815, 59.4461) (82.4178, 59.2099) (82.7383, 59.0772) (83.0724, 59.0772) knots 0 0 0 0 1 1 1 1
  line L291 (89.1392, 55.2304) -> (87.8298, 55.2531)
  spline S987 degree 3 poles (82.0642, 56.1042) (82.2201, 55.823) (82.5142, 55.6463) (82.8357, 55.6407) knots 0 0 0 0 1 1 1 1
  spline S988 degree 3 poles (76.7705, 60.4166) (76.7704, 60.8116) (76.8743, 61.1996) (77.0718, 61.5416) knots 0 0 0 0 1 1 1 1
  spline S989 degree 3 poles (83.9633, 59.4461) (84.1998, 59.6823) (84.3327, 60.0028) (84.3328, 60.337) knots 0 0 0 0 1 1 1 1
  spline S990 degree 3 poles (84.3328, 60.337) (84.3327, 60.6713) (84.1998, 60.9917) (83.9633, 61.2279) knots 0 0 0 0 1 1 1 1
  spline S991 degree 3 poles (89.8932, 53.8677) (90.0583, 54.143) (90.0642, 54.4854) (89.9087, 54.7663) knots 0 0 0 0 1 1 1 1
  spline S992 degree 3 poles (82.1815, 61.2279) (81.9453, 60.9916) (81.8125, 60.6712) (81.8126, 60.337) knots 0 0 0 0 1 1 1 1
  spline S993 degree 3 poles (95.2691, 60.5344) (95.3101, 60.4086) (95.331, 60.2771) (95.3311, 60.1448) knots 0 0 0 0 1 1 1 1
  spline S994 degree 3 poles (87.0443, 54.8164) (86.8792, 54.5411) (86.8733, 54.1987) (87.0288, 53.9178) knots 0 0 0 0 1 1 1 1
  line L292 (87.7982, 53.4537) -> (89.1082, 53.4305)
  spline S995 degree 3 poles (81.8126, 60.337) (81.8125, 60.0029) (81.9453, 59.6824) (82.1815, 59.4461) knots 0 0 0 0 1 1 1 1
  spline S996 degree 3 poles (87.5331, 38.2557) (87.2122, 38.2606) (86.9129, 38.0943) (86.7476, 37.819) knots 0 0 0 0 1 1 1 1
  spline S997 degree 3 poles (84.1452, 55.6174) (84.4663, 55.6126) (84.7656, 55.7792) (84.9307, 56.0546) knots 0 0 0 0 1 1 1 1
  spline S998 degree 3 poles (94.8118, 61.1644) (94.7047, 61.242) (94.5861, 61.3024) (94.4604, 61.3432) knots 0 0 0 0 1 1 1 1
  spline S999 degree 3 poles (83.0724, 59.0772) (83.4066, 59.0772) (83.727, 59.2099) (83.9633, 59.4461) knots 0 0 0 0 1 1 1 1
  line L293 (83.0724, 61.5969) -> (83.0724, 61.5969)
  spline S1000 degree 3 poles (83.0724, 61.5969) (83.4066, 61.5969) (83.727, 61.4642) (83.9633, 61.2279) knots 0 0 0 0 1 1 1 1
  spline S1001 degree 3 poles (84.3328, 60.337) (84.3327, 60.0028) (84.1998, 59.6823) (83.9633, 59.4461) knots 0 0 0 0 1 1 1 1
  spline S1002 degree 3 poles (89.9087, 54.7663) (90.0642, 54.4854) (90.0583, 54.143) (89.8932, 53.8677) knots 0 0 0 0 1 1 1 1
  spline S1003 degree 3 poles (95.0903, 60.8858) (95.168, 60.7788) (95.2283, 60.6602) (95.2691, 60.5344) knots 0 0 0 0 1 1 1 1
  spline S1004 degree 3 poles (94.0707, 58.8849) (93.7366, 58.8849) (93.4161, 59.0176) (93.1798, 59.2539) knots 0 0 0 0 1 1 1 1
  spline S1005 degree 3 poles (87.0443, 54.8164) (87.2095, 55.0917) (87.5088, 55.258) (87.8298, 55.2531) knots 0 0 0 0 1 1 1 1
  line L294 (87.8298, 55.2531) -> (89.1392, 55.2304)
  line L295 (87.8298, 55.2531) -> (87.8298, 55.2531)
  spline S1006 degree 3 poles (86.7476, 37.819) (86.5826, 37.5437) (86.5767, 37.2013) (86.7321, 36.9204) knots 0 0 0 0 1 1 1 1
  spline S1007 degree 3 poles (81.8126, 60.337) (81.8125, 60.6712) (81.9453, 60.9916) (82.1815, 61.2279) knots 0 0 0 0 1 1 1 1
  spline S1008 degree 3 poles (83.9633, 61.2279) (83.727, 61.4642) (83.4066, 61.5969) (83.0724, 61.5969) knots 0 0 0 0 1 1 1 1
  line L296 (79.0205, 62.6666) -> (79.0205, 62.6666)
  spline S1009 degree 3 poles (83.9633, 61.2279) (84.1998, 60.9917) (84.3327, 60.6713) (84.3328, 60.337) knots 0 0 0 0 1 1 1 1
  spline S1010 degree 3 poles (89.8932, 53.8677) (89.7282, 53.5924) (89.4291, 53.4258) (89.1082, 53.4305) knots 0 0 0 0 1 1 1 1
  spline S1011 degree 3 poles (84.9307, 56.0546) (85.0958, 56.33) (85.1017, 56.6724) (84.9462, 56.9533) knots 0 0 0 0 1 1 1 1
  spline S1012 degree 3 poles (79.0205, 58.1666) (78.6255, 58.1667) (78.2375, 58.2708) (77.8955, 58.4684) knots 0 0 0 0 1 1 1 1
  spline S1013 degree 3 poles (95.3311, 60.1448) (95.3311, 59.8107) (95.1984, 59.4902) (94.9621, 59.2539) knots 0 0 0 0 1 1 1 1
  line L297 (94.0707, 61.4052) -> (94.0707, 61.4052)
  line L298 (83.0724, 61.5969) -> (83.0724, 61.5969)
  spline S1014 degree 3 poles (93.1798, 59.2539) (92.9436, 59.4902) (92.8108, 59.8107) (92.8108, 60.1448) knots 0 0 0 0 1 1 1 1
  spline S1015 degree 3 poles (89.1082, 53.4305) (89.4291, 53.4258) (89.7282, 53.5924) (89.8932, 53.8677) knots 0 0 0 0 1 1 1 1
  spline S1016 degree 3 poles (83.9633, 59.4461) (83.727, 59.2099) (83.4066, 59.0772) (83.0724, 59.0772) knots 0 0 0 0 1 1 1 1
  line L299 (82.8357, 55.6407) -> (84.1452, 55.6174)
  spline S1017 degree 3 poles (77.8955, 58.4684) (77.5534, 58.6658) (77.2693, 58.9497) (77.0718, 59.2916) knots 0 0 0 0 1 1 1 1
  spline S1018 degree 3 poles (77.8955, 62.3653) (78.2375, 62.5628) (78.6255, 62.6667) (79.0205, 62.6666) knots 0 0 0 0 1 1 1 1
  line L300 (94.0707, 61.4052) -> (94.0707, 61.4052)
  spline S1019 degree 3 poles (94.9621, 59.2539) (94.7257, 59.0175) (94.405, 58.8848) (94.0707, 58.8849) knots 0 0 0 0 1 1 1 1
  spline S1020 degree 3 poles (87.7982, 53.4537) (87.4773, 53.4602) (87.1842, 53.637) (87.0288, 53.9178) knots 0 0 0 0 1 1 1 1
  line L301 (89.1082, 53.4305) -> (87.7982, 53.4537)
  spline S1021 degree 3 poles (86.7321, 36.9204) (86.8875, 36.6396) (87.1807, 36.4627) (87.5016, 36.4563) knots 0 0 0 0 1 1 1 1
  spline S1022 degree 3 poles (77.0718, 61.5416) (77.2693, 61.8837) (77.5534, 62.1678) (77.8955, 62.3653) knots 0 0 0 0 1 1 1 1
  spline S1023 degree 3 poles (94.4604, 61.3432) (94.5861, 61.3024) (94.7047, 61.242) (94.8118, 61.1644) knots 0 0 0 0 1 1 1 1
  spline S1024 degree 3 poles (93.1798, 61.0362) (93.4161, 61.2725) (93.7366, 61.4052) (94.0707, 61.4052) knots 0 0 0 0 1 1 1 1
  spline S1025 degree 3 poles (83.0724, 59.0772) (82.7383, 59.0772) (82.4178, 59.2099) (82.1815, 59.4461) knots 0 0 0 0 1 1 1 1
  spline S1026 degree 3 poles (87.8298, 55.2531) (87.5088, 55.258) (87.2095, 55.0917) (87.0443, 54.8164) knots 0 0 0 0 1 1 1 1
  spline S1027 degree 3 poles (89.1392, 55.2304) (89.4601, 55.224) (89.7533, 55.0471) (89.9087, 54.7663) knots 0 0 0 0 1 1 1 1
  spline S1028 degree 3 poles (77.0718, 61.5416) (76.8743, 61.1996) (76.7704, 60.8116) (76.7705, 60.4166) knots 0 0 0 0 1 1 1 1
  spline S1029 degree 3 poles (76.7705, 60.4166) (76.7704, 60.0217) (76.8743, 59.6337) (77.0718, 59.2916) knots 0 0 0 0 1 1 1 1
  spline S1030 degree 3 poles (75.5752, 64.5037) (75.2411, 64.5037) (74.9206, 64.371) (74.6843, 64.1347) knots 0 0 0 0 1 1 1 1
  spline S1031 degree 3 poles (71.5093, 56.8938) (71.3486, 56.6154) (71.0515, 56.4438) (70.73, 56.4437) knots 0 0 0 0 1 1 1 1
  spline S1032 degree 3 poles (68.6407, 56.8938) (68.4801, 57.1722) (68.4801, 57.5151) (68.6407, 57.7935) knots 0 0 0 0 1 1 1 1
  spline S1033 degree 3 poles (79.0205, 62.6666) (78.6255, 62.6667) (78.2375, 62.5628) (77.8955, 62.3653) knots 0 0 0 0 1 1 1 1
  spline S1034 degree 3 poles (76.4661, 62.3524) (76.7025, 62.5888) (76.8352, 62.9095) (76.8351, 63.2438) knots 0 0 0 0 1 1 1 1
  spline S1035 degree 3 poles (77.8955, 58.4684) (78.2375, 58.2708) (78.6255, 58.1667) (79.0205, 58.1666) knots 0 0 0 0 1 1 1 1
  spline S1036 degree 3 poles (72.0648, 62.7105) (72.1115, 62.8845) (72.1351, 63.0638) (72.1351, 63.2438) knots 0 0 0 0 1 1 1 1
  spline S1037 degree 3 poles (79.0205, 58.1666) (79.4155, 58.1667) (79.8035, 58.2708) (80.1455, 58.4684) knots 0 0 0 0 1 1 1 1
  spline S1038 degree 3 poles (76.3157, 64.2629) (76.2087, 64.3406) (76.0901, 64.4009) (75.9643, 64.4417) knots 0 0 0 0 1 1 1 1
  spline S1039 degree 3 poles (68.6407, 57.7935) (68.4801, 57.5151) (68.4801, 57.1722) (68.6407, 56.8938) knots 0 0 0 0 1 1 1 1
  spline S1040 degree 3 poles (71.5093, 57.7935) (71.67, 57.5151) (71.67, 57.1722) (71.5093, 56.8938) knots 0 0 0 0 1 1 1 1
  spline S1041 degree 3 poles (70.6081, 65.2334) (70.4343, 65.28) (70.2552, 65.3036) (70.0753, 65.3037) knots 0 0 0 0 1 1 1 1
  spline S1042 degree 3 poles (80.9687, 59.2916) (81.1663, 59.6336) (81.2704, 60.0216) (81.2705, 60.4166) knots 0 0 0 0 1 1 1 1
  spline S1043 degree 3 poles (75.5752, 61.9834) (75.9094, 61.9834) (76.2298, 62.1162) (76.4661, 62.3524) knots 0 0 0 0 1 1 1 1
  spline S1044 degree 3 poles (69.42, 58.2436) (69.0985, 58.2436) (68.8015, 58.072) (68.6407, 57.7935) knots 0 0 0 0 1 1 1 1
  spline S1045 degree 3 poles (71.5315, 64.7001) (71.4043, 64.8274) (71.261, 64.9376) (71.1052, 65.0277) knots 0 0 0 0 1 1 1 1
  spline S1046 degree 3 poles (69.42, 56.4437) (69.0985, 56.4438) (68.8015, 56.6154) (68.6407, 56.8938) knots 0 0 0 0 1 1 1 1
  spline S1047 degree 3 poles (71.5093, 56.8938) (71.67, 57.1722) (71.67, 57.5151) (71.5093, 57.7935) knots 0 0 0 0 1 1 1 1
  line L302 (69.42, 58.2436) -> (69.42, 58.2436)
  spline S1048 degree 3 poles (76.5943, 63.9844) (76.5166, 64.0912) (76.4226, 64.1852) (76.3157, 64.2629) knots 0 0 0 0 1 1 1 1
  spline S1049 degree 3 poles (72.1351, 63.2438) (72.135, 63.4237) (72.1114, 63.6029) (72.0648, 63.7766) knots 0 0 0 0 1 1 1 1
  spline S1050 degree 3 poles (77.8955, 62.3653) (77.5534, 62.1678) (77.2693, 61.8837) (77.0718, 61.5416) knots 0 0 0 0 1 1 1 1